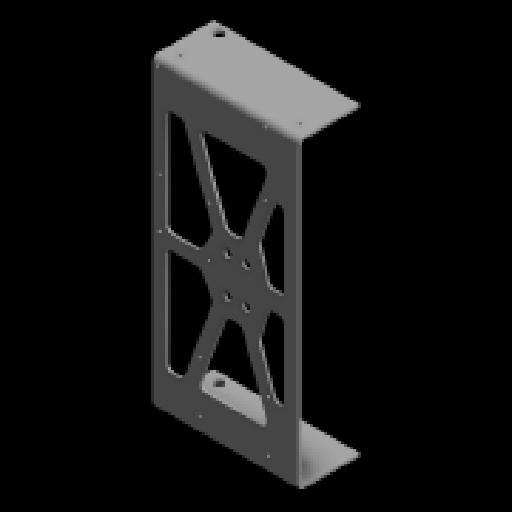
# Autodesk Inventor part: NeckMiddleBracket
Saved by Autodesk Inventor 2025.2 (Build 292293000, 293)
## iProperties
Created: 2025-09-15
Part Number: NeckMiddleBracket
Material: Generic
Document SubType Name: Sheet Metal
Designer: valer
Density: 1 g/cm^3
Sheet Metal Rule: Default
Appearance: Default
Author: valer
Autodesk Inventor part; units mm, degrees
ref_plane "YZ Plane" through (0, 0, 0) normal (1, 0, 0) x (0, 1, 0)
ref_plane "XZ Plane" through (0, 0, 0) normal (0, 1, 0) x (-1, 0, 0)
ref_plane "XY Plane" through (0, 0, 0) normal (0, 0, 1) x (1, 0, 0)
sketch "Sketch1" plane through (0, 0, 0) normal (0, 0, 1) x (1, 0, 0)
  line L0 (-128.0777, -108.501) -> (-24.0777, -108.501)
  line L1 (-24.0777, -108.501) -> (-24.0777, 108.501)
  line L2 (-24.0777, 108.501) -> (-128.0777, 108.501)
  line L3 (-128.0777, 108.501) -> (-128.0777, -108.501)
  line L4 (-122.0777, -108.501) -> (-44.6445, -108.501) construction
  line L5 (-122.0777, 108.501) -> (-44.6445, 108.501) construction
  line L6 (-36.0777, -111.549) -> (-30.0777, -111.549) construction
  point P0 (0, 0)
  dimension "d0" = 6
  measures "d0" distance from line of L1 L6.end
extrude "Plate1" add sketch "Sketch1" along normal blind 2
sketch "Sketch2" plane through (-128.0777, -106.501, 2) normal (0, -1, 0) x (1, 0, 0)
  line L0 (104, 0) -> (0, 0)
  line L1 (0, 0) -> (0, -44)
  line L2 (0, -44) -> (104, -44)
  line L3 (104, -44) -> (104, 0)
  constraints: 6 end point, 1 horizontal, 1 perpendicular, 1 vertical
edge flange "Flange1" height 44 angle 90 thickness 2 bend radius 2 thickness toward (0, -1, 0) relief straight relief width 2 relief depth 1 corner gap 2 corner form 0 edges at (-76.0777, -108.501, 0) (-76.0777, 108.501, 0) wall of the first edge with corners at (-24.0777, -106.501, 2) (-128.0777, -106.501, 2) (-128.0777, -106.501, -42) (-24.0777, -106.501, -42)
bend "Bend1"
corner "Corner1"
sketch "Sketch3" plane through (-128.0777, -108.501, -42) normal (0, -1, 0) x (1, 0, 0)
  circle A0 centre (10, 34) radius 3 construction
  circle A1 centre (10.678, 6.837) radius 3 projected
  circle A2 centre (95, 34) radius 3 construction
  circle A3 centre (10, 34) radius 1
  circle A4 centre (95, 34) radius 1
  point P0 (128.0777, 42)
  dimension "d16" = 2
  constraints: 2 centre point, 2 coincident, 1 equal radius
  measures "d16" diameter of A3
extrude "Cut1" cut sketch "Sketch3" against normal through all
sketch "Sketch5" plane through (0, 0, 2) normal (0, 0, 1) x (1, 0, 0)
  line L0 (-106.0777, -80.501) -> (-84.5831, -21.4451)
  line L1 (-84.5831, -21.4451) -> (-94.0777, -5)
  line L2 (-94.0777, -5) -> (-118.0777, -5)
  line L3 (-24.0777, -104.501) -> (-128.0777, -104.501) construction
  line L4 (-118.0777, -5) -> (-118.0777, -80.501)
  line L5 (-118.0777, -80.501) -> (-106.0777, -80.501)
  line L6 (-128.0777, 104.501) -> (-24.0777, 104.501) construction
  line L7 (-24.0777, 0) -> (-128.0777, 0) construction
  line L8 (-128.0777, 104.501) -> (-128.0777, -104.501) construction
  line L9 (-106.0777, 80.501) -> (-84.5831, 21.4451)
  line L10 (-84.5831, 21.4451) -> (-94.0777, 5)
  line L11 (-94.0777, 5) -> (-118.0777, 5)
  line L12 (-118.0777, 5) -> (-118.0777, 80.501)
  line L13 (-118.0777, 80.501) -> (-106.0777, 80.501)
  circle A0 centre (-74.3541, 13.095) radius 3 projected
  circle A1 centre (-60.9541, 13.095) radius 3 projected
  circle A2 centre (-60.9541, -13.095) radius 3 projected
  circle A3 centre (-74.3541, -13.095) radius 3 projected
  line L14 (-24.0777, 104.501) -> (-24.0777, -104.501) construction
  line L15 (-75.646, -26.1287) -> (-95.4359, -80.501)
  line L16 (-95.4359, -80.501) -> (-44.7195, -80.501)
  line L17 (-44.7195, -80.501) -> (-64.5094, -26.1287)
  line L18 (-64.5094, -26.1287) -> (-75.646, -26.1287)
  line L19 (-52.5436, -29.7663) -> (-45.2143, -6.5168)
  line L20 (-45.2143, -6.5168) -> (-34.0777, -6.5168)
  line L21 (-34.0777, -6.5168) -> (-34.0777, -80.501)
  line L22 (-34.0777, -80.501) -> (-52.5436, -29.7663)
  line L23 (-44.7195, -80.501) -> (-34.0777, -80.501) construction
  line L24 (-84.5831, -21.4451) -> (-75.646, -26.1287) construction
  line L25 (-75.646, 26.1287) -> (-95.4359, 80.501)
  line L26 (-95.4359, 80.501) -> (-44.7195, 80.501)
  line L27 (-44.7195, 80.501) -> (-64.5094, 26.1287)
  line L28 (-64.5094, 26.1287) -> (-75.646, 26.1287)
  line L29 (-52.5436, 29.7663) -> (-45.2143, 6.5168)
  line L30 (-45.2143, 6.5168) -> (-34.0777, 6.5168)
  line L31 (-34.0777, 6.5168) -> (-34.0777, 80.501)
  line L32 (-34.0777, 80.501) -> (-52.5436, 29.7663)
  point P0 (0, 0)
  point P1 (-112.0777, -80.501)
  dimension "d17" = 10
  dimension "d18" = 24
  dimension "d19" = 10
  dimension "d20" = 120
  dimension "d21" = 12
  dimension "d22" = 130
  dimension "d23" = 24
  dimension "d24" = 70
  dimension "d25" = 70
  dimension "d26" = 10
  dimension "d27" = 10
  dimension "d28" = 10
  dimension "d29" = 13.0337
  dimension "d30" = 13.0337
  dimension "d31" = 13.0337
  dimension "d32" = 6.5168
  dimension "d33" = 152.343
  constraints: 58 end point, 13 symmetric about line, 6 parallel, 3 horizontal, 3 midpoint, 2 perpendicular, 1 collinear
  measures "d17" distance between parallel lines of L8 L4
  measures "d18" distance from line of point (-112.078, -80.501) L3
  measures "d19" distance between parallel lines of L11 L2
  measures "d20" angle of L2 L1
  measures "d21" distance of L4.end L0.start
  measures "d22" angle of L1 L0
  measures "d23" distance of L1.end L2.end
  measures "d24" angle of L15 L16
  measures "d25" angle of L17 L16
  measures "d26" distance between parallel lines of L14 L21
  measures "d27" distance between parallel lines of L0 L15
  measures "d28" distance between parallel lines of L22 L17
  measures "d29" distance from line of L1 A3.centre
  measures "d30" distance from line of A3.centre L18
  measures "d31" distance from line of A2.centre L19
  measures "d32" distance between parallel lines of L7 L20
  measures "d33" angle of L24 L18
extrude "Cut3" cut sketch "Sketch5" against normal blind 2
fillet "Fillet1" radius 4 26 edges at (-118.0777, -80.501, 1) (-106.0777, -80.501, 1) (-118.0777, -5, 1) (-84.5831, -21.4451, 1) (-94.0777, -5, 1) (-118.0777, 5, 1) (-118.0777, 80.501, 1) (-94.0777, 5, 1) (-84.5831, 21.4451, 1) (-106.0777, 80.501, 1) (-95.4359, -80.501, 1) (-44.7195, -80.501, 1) (-64.5094, -26.1287, 1) (-75.646, -26.1287, 1) (-95.4359, 80.501, 1) (-75.646, 26.1287, 1) (-64.5094, 26.1287, 1) (-44.7195, 80.501, 1) (-52.5436, 29.7663, 1) (-45.2143, 6.5168, 1) (-34.0777, 6.5168, 1) (-34.0777, 80.501, 1) (-34.0777, -80.501, 1) (-52.5436, -29.7663, 1) (-45.2143, -6.5168, 1) (-34.0777, -6.5168, 1)
sketch "MountHoles" plane through (0, 0, 2) normal (0, 0, 1) x (1, 0, 0)
  circle A0 centre (-122.5777, 2.9262) radius 1.6 construction
  circle A1 centre (-122.5777, 38.4262) radius 1.6 construction
  circle A2 centre (-87.0777, 38.4262) radius 1.6 construction
  circle A3 centre (-87.0777, 2.9262) radius 1.6 construction
  circle A4 centre (-94.0777, -96.501) radius 1.25 construction
  circle A5 centre (-94.0777, -60.501) radius 1.25 construction
  circle A6 centre (-45.0777, -60.501) radius 1.25 construction
  circle A7 centre (-45.0777, -96.501) radius 1.25 construction
  circle A8 centre (-123.5677, 104.5662) radius 1.65 construction
  circle A9 centre (-47.6177, 104.5662) radius 1.65 construction
  circle A10 centre (-47.6177, 59.4362) radius 1.65 construction
  circle A11 centre (-122.5777, 38.4262) radius 1
  circle A12 centre (-123.5677, 104.5662) radius 1
  circle A13 centre (-47.6177, 104.5662) radius 1
  circle A14 centre (-47.6177, 59.4362) radius 1
  circle A15 centre (-87.0777, 38.4262) radius 1
  circle A16 centre (-94.0777, -96.501) radius 1
  circle A17 centre (-94.0777, -60.501) radius 1
  circle A18 centre (-45.0777, -96.501) radius 1
  circle A19 centre (-45.0777, -60.501) radius 1
  circle A20 centre (-122.5777, 2.9262) radius 1
  circle A21 centre (-87.0777, 2.9262) radius 1
  point P0 (0, 0)
  dimension "d37" = 2
  dimension "d38" = 2
  dimension "d39" = 2
  dimension "d40" = 2
  dimension "d41" = 2
  dimension "d42" = 2
  dimension "d43" = 2
  dimension "d44" = 2
  dimension "d45" = 2
  dimension "d46" = 2
  dimension "d47" = 2
  constraints: 11 centre point, 11 coincident
  measures "d37" diameter of A11
  measures "d38" diameter of A12
  measures "d39" diameter of A13
  measures "d40" diameter of A14
  measures "d41" diameter of A15
  measures "d42" diameter of A16
  measures "d43" diameter of A17
  measures "d44" diameter of A18
  measures "d45" diameter of A19
  measures "d46" diameter of A20
  measures "d47" diameter of A21
extrude "Cut4" cut sketch "MountHoles" against normal blind 2
equation "\"d12\" = Thickness"
equation "\"d25\" = d24"
equation "\"d26\" = d17"
equation "\"d27\" = d17"
equation "\"d28\" = d17"
equation "\"d30\" = d29"
equation "\"d31\" = d29"
equation "\"d32\" = 0.5 * d29"
equation "\"d34\" = Thickness"
equation "\"d48\" = Thickness"
equation "\"d1\" = Thickness"
equation "\"d2\" = BendReliefWidth"
equation "\"d3\" = BendReliefDepth"
equation "\"d4\" = MinimumRemnant"
equation "\"d5\" = TransitionRadius"
equation "\"d8\" = BendRadius"
equation "\"d9\" = CornerReliefSize"
equation "\"d10\" = GapSize"
equation "\"d11\" = JacobiRadiusSize"
equation "\"BendRadius\" = Thickness"
equation "\"BendReliefWidth\" = Thickness"
equation "\"BendReliefDepth\" = 0.5 * Thickness"
equation "\"CornerReliefSize\" = 4 * Thickness"
equation "\"MinimumRemnant\" = 2 * Thickness"
equation "\"TransitionRadius\" = BendRadius"
equation "\"JacobiRadiusSize\" = BendRadius"
equation "\"GapSize\" = Thickness"
equation "\"Thickness\" = 2"
body "Solid1"
